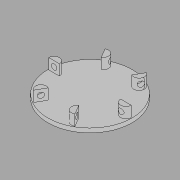
# Autodesk Inventor part: base
Saved by Autodesk Inventor 2020 (Build 240168000, 168)
## iProperties
Created: 2020-12-28
Part Number: base
Material: Generic
Document SubType Name: Modeling
Designer: freyja
Density: 1 g/cm^3
Appearance: Default
Author: freyja
Autodesk Inventor part; units mm, degrees
ref_plane "YZ Plane" through (0, 0, 0) normal (1, 0, 0) x (0, 1, 0)
ref_plane "XZ Plane" through (0, 0, 0) normal (0, 1, 0) x (-1, 0, 0)
ref_plane "XY Plane" through (0, 0, 0) normal (0, 0, 1) x (1, 0, 0)
sketch "Sketch1" plane through (0, 0, 0) normal (0, 1, 0) x (-1, 0, 0)
  circle A0 centre (0, 0) radius 50
  dimension "d0" = 100
  constraints: 1 centre point, 1 coincident
  measures "d0" diameter of A0
extrude "Extrusion1" add sketch "Sketch1" along normal blind 5
sketch "Sketch2" plane through (0, 5, 0) normal (0, 1, 0) x (1, 0, 0)
  circle A0 centre (-42.7717, 0) radius 6.35
  point P0 (0, 0)
  dimension "d3" = 12.7
  constraints: 1 centre point
  measures "d3" diameter of A0
extrude "Extrusion2" add sketch "Sketch2" along normal blind 12.7
sketch "Sketch3" plane through (-42.7717, 17.7, 0) normal (0, 1, 0) x (1, 0, 0)
  circle A0 centre (0, 0) radius 6.35 projected
  circle A1 centre (0, 0) radius 6.35 projected
  line L0 (-6.35, 0) -> (6.35, 0)
  point P0 (42.7717, 0)
  constraints: 2 end point, 2 point on circle, 1 horizontal, 1 midpoint
extrude "Extrusion3" cut sketch "Sketch3" against normal blind 12.7 contours A0 L0 picked at (-1.2024, -1.742)
sketch "Sketch4" plane through (-49.1217, 17.7, 0) normal (0, 0, 1) x (1, 0, 0)
  line L0 (0, 0) -> (12.7, 0) projected
  line L1 (12.7, 0) -> (12.7, -12.7) projected
  point P0 (49.1217, -17.7)
  point P1 (6.35, -6.35)
  dimension "d8" = 6.35
  dimension "d9" = 12.7
  dimension "d10" = 6.35
  measures "d8" distance from line of L0 point (6.35, -6.35)
  measures "d9" distance of L0.start L0.end
  measures "d10" distance from line of L1 point (6.35, -6.35)
hole "Hole1" at (-42.7717, 11.35, 0) direction (0, 0, -1) diameter 6.5278 end through all clearance for "Flat Head Machine Screw (82)" size "1/4" standard "Ansi Unified Screw Threads"
pattern_circular "Circular Pattern1" count 6 over 360 about axis through (0, -10, 0) along (0, 1, 0) of "Hole1", "Extrusion2", "Extrusion3"
equation "\"d10\" = 0.5 * d9"
body "Solid1"
